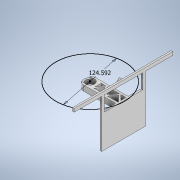
# Autodesk Inventor part: Tower
Saved by Autodesk Inventor 2022 (Build 260153000, 153)
## iProperties
Created: 2023-03-16
Part Number: Tower
Material: Generic
Document SubType Name: Modeling
Designer: Jacki
Density: 1 g/cm^3
Appearance: Default
Author: Jacki
Autodesk Inventor part; units mm, degrees
ref_plane "YZ Plane" through (0, 0, 0) normal (1, 0, 0) x (0, 1, 0)
ref_plane "XZ Plane" through (0, 0, 0) normal (0, 1, 0) x (-1, 0, 0)
ref_plane "XY Plane" through (0, 0, 0) normal (0, 0, 1) x (1, 0, 0)
sketch "Sketch1" plane through (0, 0, 0) normal (0, 1, 0) x (-1, 0, 0)
  line L0 (-122.594, 12.25) -> (-122.594, -12.2908)
  line L1 (-61.296, -11.2083) -> (-61.296, 11.2917)
  line L2 (0, 0) -> (-13.1, 0)
  line L3 (-61.296, 0) -> (-63.296, 0)
  circle A0 centre (0, 0.0417) radius 8.25
  arc A1 (0, -11.2083) -> (0, 11.2917) centre (0, 0.0417) ccw
  line L4 (0, -11.2083) -> (-61.296, -11.2083)
  line L5 (0, 11.2917) -> (-61.296, 11.2917)
  dimension "d24" = 61.296
  dimension "d28" = 16.5
  dimension "d30" = 3
  constraints: 12 end point, 2 centre point, 2 horizontal, 2 perpendicular, 2 point on circle, 2 tangent, 1 coincident, 1 point on line
  measures "d24" distance from line of point (0, 0) L1
  measures "d28" diameter of A0
  measures "d30" radial gap between concentric circles of A0 A1
extrude "Extrusion1" add sketch "Sketch1" along normal blind 10
sketch "Sketch3" plane through (0, 10, 0) normal (0, 1, 0) x (1, 0, 0)
  line L0 (8.1183, -12.2504) -> (8.1163, 12.2496)
  line L1 (13.1167, 7.25) -> (13.1179, -7.25)
  line L2 (39.1319, -7.25) -> (47.9899, 4.2277)
  line L3 (36.5087, -5.7388) -> (46.5328, 7.25)
  line L4 (49.2102, 7.25) -> (62.1991, -5.7388)
  line L5 (13.1179, -7.25) -> (61.3127, -7.25)
  line L6 (61.296, -11.2917) -> (61.296, 11.2083) projected
  line L7 (13.1167, 7.25) -> (61.3127, 7.25)
  line L8 (61.3127, -7.25) -> (61.3127, 7.25)
  line L9 (47.9899, 4.2277) -> (59.4676, -7.25)
  line L10 (61.296, -9.1202) -> (61.4899, -9.3141)
  line L11 (49.2102, 7.25) -> (61.296, -4.8775)
  line L12 (13.1179, -7.25) -> (21.1056, -7.25)
  line L13 (21.1056, 7.25) -> (13.1179, 7.25)
  line L14 (13.1179, 7.25) -> (13.1179, -7.25)
  line L15 (24.1056, -7.25) -> (33.7772, -7.25)
  line L16 (21.1057, 5.5674) -> (21.1056, 5.5673)
  line L17 (23.5198, 7.25) -> (23.5198, -7.25)
  line L18 (36.5087, -5.7388) -> (35.3424, -7.25)
  line L19 (11.5087, -5.7388) -> (10.3424, -7.25)
  line L20 (11.5087, -5.7388) -> (21.5328, 7.25)
  line L21 (14.1319, -7.25) -> (22.9899, 4.2277)
  line L22 (22.9899, 4.2277) -> (34.4676, -7.25)
  line L23 (24.2102, 7.25) -> (36.296, -4.8775)
  line L24 (24.2102, 7.25) -> (37.1991, -5.7388)
  line L25 (36.3127, -7.25) -> (36.3127, 7.25)
  line L26 (36.296, -9.1202) -> (36.4899, -9.3141)
  point P0 (0, 0)
  point P1 (0, 0)
  point P2 (61.297, -12.25)
  point P3 (61.295, 12.2704)
  point P4 (62.1991, -5.7388)
  point P5 (61.2954, 7.25)
  point P6 (61.296, -4.8358)
  point P7 (61.296, -7.25)
  point P8 (61.296, 7.25)
  point P9 (13.1179, -1.906)
  point P10 (36.8094, -5.3492)
  point P11 (13.1179, -3.6537)
  point P12 (21.5328, 7.25)
  dimension "d9" = 5
  dimension "d53" = 25
  constraints: 52 end point, 10 point on line, 3 horizontal, 2 parallel, 1 collinear, 1 perpendicular, 1 vertical, 24 other
  measures "d9" distance between parallel lines of L0 L1
  measures "d53" distance of L18.end L19.end
extrude "Extrusion2" cut sketch "Sketch3" against normal blind 10 contours L7 L20 L1 | L21 L22 L17 L5 | L7 L25 L24 | L22 L5 L17 | L7 L3 L24 L25 | L7 L6 L4 | L2 L9 L5
sketch "Sketch7" plane through (0, 10, 0) normal (0, 1, 0) x (1, 0, 0)
  circle A0 centre (0, 0) radius 62.296
  dimension "d20" = 124.592
  constraints: 1 centre point, 1 coincident
  measures "d20" diameter of A0
sketch "Sketch8" plane through (61.296, 0, 12.25) normal (1, 0, 0) x (0, 0, -1)
  line L0 (-27.75, 0) -> (52.25, 0)
  line L1 (52.25, 0) -> (52.25, 10)
  line L2 (52.25, 10) -> (-27.75, 10)
  line L3 (-27.75, 10) -> (-27.75, 0)
  line L4 (-27.75, 0) -> (52.25, 10) construction
  line L5 (52.25, 0) -> (-27.75, 10) construction
  line L6 (52.25, 10) -> (-27.75, 10)
  line L7 (-27.75, 10) -> (-27.75, -50)
  line L8 (-27.75, -50) -> (52.25, -50)
  line L9 (52.25, -50) -> (52.25, 10)
  line L10 (52.25, 10) -> (47.25, 10)
  line L11 (47.25, 10) -> (47.25, 37)
  line L12 (-27.75, 10) -> (52.25, 10)
  line L13 (-27.75, 37) -> (-27.75, 10)
  line L14 (-27.75, 10) -> (-22.75, 10)
  line L15 (-22.75, 10) -> (-22.75, 37)
  line L16 (-22.75, 37) -> (47.25, 37)
  line L17 (52.25, 43) -> (-27.75, 43)
  line L18 (-30.75, 10.375) -> (-30.75, 10)
  line L19 (-77.7917, 37) -> (-77.7917, 43)
  line L20 (-77.7917, 43) -> (102.2083, 43)
  line L21 (102.2083, 43) -> (102.2083, 37)
  line L22 (102.2083, 37) -> (-77.7917, 43) construction
  line L23 (-77.7917, 37) -> (102.2083, 43) construction
  line L24 (-27.75, 37) -> (-77.7917, 37)
  line L25 (52.25, 10) -> (52.25, 37)
  line L26 (52.25, 37) -> (52.25, 10)
  line L27 (102.2083, 37) -> (52.25, 37)
  line L28 (47.25, 37) -> (-22.75, 37)
  line L29 (23.4583, 10) -> (0.9583, 10) projected
  line L30 (12.2083, 10) -> (12.2083, 37)
  point P0 (12.25, 0)
  point P1 (47.25, 10)
  point P2 (-57.7845, 37.6669)
  point P3 (47.25, 10)
  point P4 (12.2083, 40)
  dimension "d21" = 80
  dimension "d34" = 60
  dimension "d41" = 5
  dimension "d44" = 180
  dimension "d58" = 0
  constraints: 60 end point, 11 perpendicular, 10 parallel, 4 point on line, 3 horizontal, 3 midpoint, 1 vertical
  measures "d21" distance of L0.start L0.end
  measures "d34" distance of L6.end L7.end
  measures "d41" distance of L6.end L14.end
  measures "d44" distance of L21.end L19.start
  measures "d58" distance from line of L30 point (12.208, 40)
extrude "Extrusion4" add sketch "Sketch8" against normal blind 3 contours L3 L2 L1 L0 | L0 L9 L8 L7 | L13 L24 L19 L20 L17 L21 L27 L25 L2 L11 L16 L15
sketch "Sketch11" plane through (0, 10, 0) normal (0, 1, 0) x (1, 0, 0)
  circle A0 centre (0, -0.0417) radius 8.25 projected
  line L0 (-3.0682, -7.7) -> (-14.6805, -7.7)
  line L1 (-14.6805, -7.7) -> (-14.6805, 7.7)
  line L2 (-14.6805, 7.7) -> (-3.0682, 7.7)
  line L3 (-3.0682, 7.7) -> (-3.0682, 7.6165)
  line L4 (-3.0682, -7.7) -> (0, -7.7)
  line L5 (0, -7.7) -> (0, -0.0417)
  line L6 (0, -0.0417) -> (0, 7.7)
  line L7 (0, 7.7) -> (-3.0682, 7.7)
  point P0 (0, 0)
  point P1 (-4.1158, 7.1083)
  point P2 (-2.8509, 7.7)
  dimension "d39" = 15.4
  dimension "d40" = 7.7
  constraints: 16 end point, 3 perpendicular, 2 horizontal, 2 parallel, 2 point on circle, 1 point on line
  measures "d39" distance between parallel lines of L2 L0
  measures "d40" distance from line of point (0, 0) L0
extrude "Extrusion6" cut sketch "Sketch11" against normal blind 2 contours L3 L7 A0 | A0 L0 L1 L2 L3 | L4 L5 L6 L7 A0 picked at (0.9906, 5.1042)
sketch "Sketch12" plane through (58.296, 0, 12.25) normal (-1, 0, 0) x (0, 0, 1)
  point P0 (-12.25, 0)
sketch "Sketch14" plane through (58.296, 0, 12.25) normal (-1, 0, 0) x (0, 0, 1)
  line L0 (-102.2083, 43) -> (77.7917, 43) projected
  line L1 (22.75, 37) -> (-47.25, 37) projected
  line L2 (-12.2083, 43) -> (-16.882, 38.3262)
  line L3 (-12.2083, 43) -> (-5.5985, 43) construction
  line L4 (-16.882, 38.3262) -> (-18.25, 37)
  line L5 (-12.2083, 43) -> (-7.0615, 37.8533)
  line L6 (-12.2083, 43) -> (-4.9297, 43) construction
  line L7 (-7.0615, 37.8533) -> (-6.2083, 37)
  line L8 (-6.2083, 37) -> (-18.25, 37)
  point P0 (-12.25, 0)
  dimension "d45" = 135
  dimension "d46" = 45
  constraints: 14 end point, 3 point on line, 2 equal length, 2 horizontal, 1 midpoint
  measures "d45" angle of L2 L3
  measures "d46" angle of L5 L6
extrude "Extrusion7" add sketch "Sketch14" along normal blind 5
body "Solid1"
